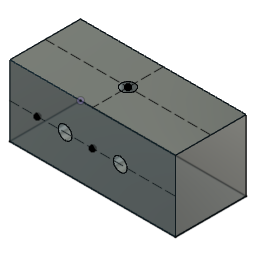
BearingTensionerBlock v10 (Autodesk Fusion 360 design; units mm, degrees)
Autodesk Fusion 360 part; units mm, degrees
sketch "Sketch1" plane through (0, 0, 0) normal (0, 1, 0) x (1, 0, 0)
  line L0 (0, 0) -> (30, 0)
  line L1 (30, 0) -> (30, -12.8)
  line L2 (30, -12.8) -> (0, -12.8)
  line L3 (0, -12.8) -> (0, 0)
  dimension "d1" = 30
  dimension "d2" = 12.8
  constraint horizontal L0
  constraint vertical L1
  constraint horizontal L2
  constraint vertical L3
  constraint coincident L0.start L3.end
  measures "d1" distance of L0.start L0.end
  measures "d2" distance of L0.start L2.end
extrude "Extrude1" add sketch "Sketch1" along normal blind 12.8
sketch "Sketch2" plane through (0, 12.8, 0) normal (0, 1, 0) x (-1, 0, 0)
  line L0 (0, 12.8) -> (-30, 12.8)
  line L1 (-30, 12.8) -> (-30, 0)
  line L2 (-30, 0) -> (0, 0)
  line L3 (0, 0) -> (0, 12.8)
  line L4 (-15, 0) -> (-15, 12.8) construction
  line L5 (0, 6.4) -> (-30, 6.4) construction
  point P0 (-15, 6.4)
  constraint midpoint L2 L4.start
  constraint midpoint L0 L4.end
  constraint midpoint L3 L5.start
  constraint midpoint L1 L5.end
  constraint midpoint L4 P0
hole "Hole1" at (15, 12.8, 6.4) direction (0, -1, 0) diameter 2.5 end through all
sketch "Sketch3" plane through (0, 0, 12.8) normal (0, 0, 1) x (1, 0, 0)
  line L0 (0, 0) -> (30, 0)
  line L1 (30, 0) -> (30, 12.8)
  line L2 (30, 12.8) -> (0, 12.8)
  line L3 (0, 12.8) -> (0, 0)
  line L4 (0, 6.4) -> (30, 6.4) construction
  point P0 (5, 6.4)
  point P1 (15, 6.4)
  dimension "d8" = 10
  dimension "d9" = 5
  constraint midpoint L3 L4.start
  constraint midpoint L1 L4.end
  constraint coincident L4 P0
  constraint coincident L4 P1
  measures "d8" distance of P0 P1
  measures "d9" distance of L3 P0
hole "Hole2" at (10, 6.4, 12.8) direction (0, 0, -1) diameter 2.5 end through all
hole "Hole3" at (20, 6.4, 12.8) direction (0, 0, -1) diameter 2.5 end through all
